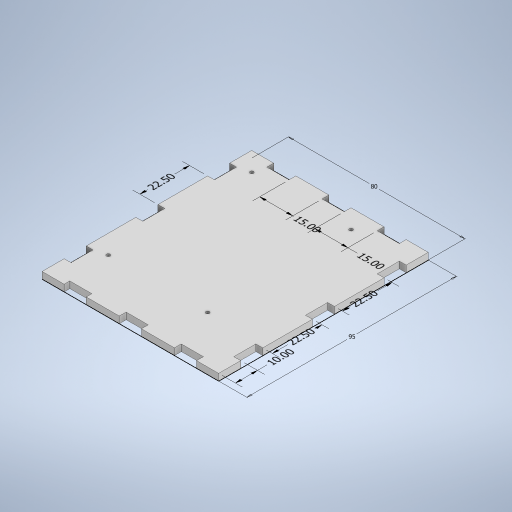
# Autodesk Inventor part: Fundo
Saved by Autodesk Inventor 2024 (Build 280153000, 153)
## iProperties
Created: 2023-11-29
Part Number: Fundo
Material: Genérico
Document SubType Name: Modeling
Designer: caiot
Density: 1 g/cm^3
Appearance: Padrão
Author: caiot
Autodesk Inventor part; units mm, degrees
ref_plane "YZ Plane" through (0, 0, 0) normal (1, 0, 0) x (0, 1, 0)
ref_plane "XZ Plane" through (0, 0, 0) normal (0, 1, 0) x (-1, 0, 0)
ref_plane "XY Plane" through (0, 0, 0) normal (0, 0, 1) x (1, 0, 0)
sketch "Fundo" plane through (0, 0, 0) normal (0, 1, 0) x (-1, 0, 0)
  line L0 (0, 0) -> (-80, 0)
  line L1 (-80, 0) -> (-80, -95)
  line L2 (-80, -95) -> (0, -95)
  line L3 (0, -95) -> (0, 0)
  dimension "d0" = 80
  dimension "d1" = 95
  constraints: 8 end point, 2 parallel, 1 horizontal, 1 perpendicular
  measures "d0" distance of L2.end L1.end
  measures "d1" distance of L1.end L0.end
extrude "Extrusão1" add sketch "Fundo" along normal blind 3
sketch "Esboço3" plane through (0, 3, 0) normal (0, 1, 0) x (1, 0, 0)
  line L0 (10, -0.55) -> (20, -0.55)
  line L1 (20, -0.55) -> (20, 2.55)
  line L2 (20, 2.55) -> (10, 2.55)
  line L3 (10, 2.55) -> (10, -0.55)
  line L4 (0, 0) -> (80, 0) projected
  line L5 (70, 0) -> (60, 0)
  line L6 (60, 0) -> (60, 3.1)
  line L7 (60, 3.1) -> (70, 3.1)
  line L8 (70, 3.1) -> (70, 0)
  line L9 (35, 0) -> (45, 0)
  line L10 (45, 0) -> (45, 3.1)
  line L11 (45, 3.1) -> (35, 3.1)
  line L12 (35, 3.1) -> (35, 0)
  line L13 (80, 95) -> (0, 95) projected
  line L14 (10, 95) -> (20, 95)
  line L15 (20, 95) -> (20, 91.9)
  line L16 (20, 91.9) -> (10, 91.9)
  line L17 (10, 91.9) -> (10, 95)
  line L18 (35, 95) -> (45, 95)
  line L19 (45, 95) -> (45, 91.9)
  line L20 (45, 91.9) -> (35, 91.9)
  line L21 (35, 91.9) -> (35, 95)
  line L22 (60, 95) -> (70, 95)
  line L23 (70, 95) -> (70, 91.9)
  line L24 (70, 91.9) -> (60, 91.9)
  line L25 (60, 91.9) -> (60, 95)
  line L26 (80, 0) -> (80, 95) projected
  line L27 (0, 95) -> (0, 0) projected
  point P0 (10, 1)
  point P1 (60, 1.55)
  point P2 (20, 1)
  point P3 (35, 1.55)
  point P4 (10, 93.45)
  point P5 (70, 93.45)
  point P6 (60, 93.45)
  point P7 (45, 93.45)
  point P8 (45, 1.55)
  point P9 (35, 93.45)
  point P10 (20, 93.45)
  point P11 (20, 95)
  point P12 (45, 0)
  point P13 (60, 0)
  point P14 (70, 1.55)
  dimension "d4" = 10
  dimension "d5" = 3.1
  dimension "d7" = 10
  dimension "d8" = 3.1
  dimension "d10" = 10
  dimension "d11" = 3.1
  dimension "d18" = 10
  dimension "d19" = 3.1
  dimension "d20" = 10
  dimension "d21" = 3.1
  dimension "d22" = 10
  dimension "d23" = 3.1
  dimension "d30" = 10
  dimension "d113" = 10
  dimension "d114" = 10
  dimension "d115" = 15
  dimension "d116" = 15
  dimension "d117" = 40
  dimension "d118" = 15
  dimension "d119" = 15
  dimension "d120" = 10
  constraints: 48 end point, 12 midpoint, 12 parallel, 6 horizontal, 6 perpendicular, 3 point on line, 3 other
  measures "d4" distance of L2.end L1.end
  measures "d5" distance of L1.end L0.end
  measures "d7" distance of L6.end L7.end
  measures "d8" distance of L5.end L6.end
  measures "d10" distance of L11.end L10.end
  measures "d11" distance of L10.end L9.end
  measures "d18" distance of L15.end L16.end
  measures "d19" distance of L14.end L15.end
  measures "d20" distance of L19.end L20.end
  measures "d21" distance of L18.end L19.end
  measures "d22" distance of L23.end L24.end
  measures "d23" distance of L22.end L23.end
  measures "d30" horizontal distance of L13.end point (10, 93.45)
  measures "d113" distance from line of L26 point (70, 1.55)
  measures "d114" distance from line of L27 point (10, 1)
  measures "d115" horizontal distance of point (35, 1.55) point (20, 1)
  measures "d116" distance of point (60, 1.55) point (45, 1.55)
  measures "d117" horizontal distance of point (20, 1) L6.end
  measures "d118" distance of point (35, 93.45) point (20, 93.45)
  measures "d119" distance of point (60, 93.45) point (45, 93.45)
  measures "d120" distance from line of L26 point (70, 93.45)
extrude "Extrusão2" cut sketch "Esboço3" against normal blind 10 contours L3 L4 L1 L0 | L3 L2 L1 L4 | L12 L11 L10 L4 | L13 L15 L16 L17 | L6 L7 L8 L4 | L13 L19 L20 L21 | L13 L23 L24 L25
sketch "Esboço4" plane through (0, 3, 0) normal (0, 1, 0) x (1, 0, 0)
  line L0 (0, 95) -> (0, 0) projected
  line L1 (0, 10) -> (3.1, 10)
  line L2 (3.1, 10) -> (3.1, 20)
  line L3 (3.1, 20) -> (0, 20)
  line L4 (0, 20) -> (0, 10)
  line L5 (0, 85) -> (3.1, 85)
  line L6 (3.1, 85) -> (3.1, 75)
  line L7 (3.1, 75) -> (0, 75)
  line L8 (0, 75) -> (0, 85)
  line L9 (0, 42.5) -> (3.1, 42.5)
  line L10 (3.1, 42.5) -> (3.1, 52.5)
  line L11 (3.1, 52.5) -> (0, 52.5)
  line L12 (0, 52.5) -> (0, 42.5)
  line L13 (10, 95) -> (0, 95) projected
  line L14 (80, 0) -> (80, 95) projected
  line L15 (80, 10) -> (76.9, 10)
  line L16 (76.9, 10) -> (76.9, 20)
  line L17 (76.9, 20) -> (80, 20)
  line L18 (80, 20) -> (80, 10)
  line L19 (80, 42.5) -> (76.9, 42.5)
  line L20 (76.9, 42.5) -> (76.9, 52.5)
  line L21 (76.9, 52.5) -> (80, 52.5)
  line L22 (80, 52.5) -> (80, 42.5)
  line L23 (80, 75) -> (76.9, 75)
  line L24 (76.9, 75) -> (76.9, 85)
  line L25 (76.9, 85) -> (80, 85)
  line L26 (80, 85) -> (80, 75)
  line L27 (70, 0) -> (80, 0) projected
  line L28 (80, 95) -> (70, 95) projected
  point P0 (1.55, 10)
  point P1 (1.55, 85)
  point P2 (1.55, 75)
  point P3 (1.55, 52.5)
  point P4 (1.55, 20)
  point P5 (78.45, 10)
  point P6 (78.45, 85)
  point P7 (78.45, 52.5)
  point P8 (78.45, 75)
  point P9 (80, 85)
  point P10 (0, 75)
  point P11 (0, 52.5)
  point P12 (0, 20)
  point P13 (78.45, 42.5)
  point P14 (78.45, 20)
  dimension "d44" = 3.1
  dimension "d45" = 10
  dimension "d46" = 10
  dimension "d47" = 3.1
  dimension "d48" = 10
  dimension "d49" = 10
  dimension "d50" = 10
  dimension "d51" = 22.5
  dimension "d53" = 3.1
  dimension "d54" = 10
  dimension "d55" = 3.1
  dimension "d56" = 10
  dimension "d57" = 3.1
  dimension "d58" = 10
  dimension "d59" = 10
  dimension "d60" = 10
  dimension "d61" = 22.5
  dimension "d64" = 22.5
  dimension "d130" = 55
  constraints: 48 end point, 12 parallel, 11 midpoint, 7 point on line, 6 horizontal, 6 perpendicular
  measures "d44" distance of L3.end L2.end
  measures "d45" distance of L2.end L1.end
  measures "d46" distance of L5.end L6.end
  measures "d47" distance of L11.end L10.end
  measures "d48" distance of L10.end L9.end
  measures "d49" vertical distance of L0.end point (1.55, 10)
  measures "d50" distance from line of L13 point (1.55, 85)
  measures "d51" distance of point (1.55, 75) point (1.55, 52.5)
  measures "d53" distance of L16.end L17.end
  measures "d54" distance of L15.end L16.end
  measures "d55" distance of L20.end L21.end
  measures "d56" distance of L19.end L20.end
  measures "d57" distance of L24.end L25.end
  measures "d58" distance of L23.end L24.end
  measures "d59" distance from line of L27 point (78.45, 10)
  measures "d60" distance from line of point (78.45, 85) L28
  measures "d61" distance of point (78.45, 52.5) point (78.45, 75)
  measures "d64" distance of point (78.45, 42.5) point (78.45, 20)
  measures "d130" distance of point (78.45, 20) point (78.45, 75)
extrude "Extrusão3" cut sketch "Esboço4" against normal blind 10
sketch "Esboço6" plane through (0, 3, 0) normal (0, 1, 0) x (1, 0, 0)
  line L0 (8.6, 86.4) -> (53.6, 86.4)
  line L1 (53.6, 86.4) -> (53.6, 21.4)
  line L2 (53.6, 21.4) -> (8.6, 21.4)
  line L3 (8.6, 21.4) -> (8.6, 86.4)
  line L4 (3.1, 85) -> (3.1, 75) projected
  line L5 (20, 91.9) -> (10, 91.9) projected
  circle A0 centre (53.6, 86.4) radius 0.8
  circle A1 centre (53.6, 21.4) radius 0.8
  circle A2 centre (8.6, 21.4) radius 0.8
  circle A3 centre (8.6, 86.4) radius 0.8
  point P0 (0, 0)
  point P1 (3.1, 80)
  point P2 (15, 91.9)
  dimension "d134" = 65
  dimension "d135" = 45
  dimension "d136" = 5.5
  dimension "d137" = 5.5
  dimension "d138" = 1.6
  dimension "d139" = 1.6
  dimension "d140" = 1.6
  dimension "d141" = 1.6
  constraints: 8 end point, 4 centre point, 4 coincident, 2 midpoint, 2 parallel, 1 horizontal, 1 perpendicular
  measures "d134" distance of L0.end L1.end
  measures "d135" distance between parallel lines of L3 L1
  measures "d136" distance from line of point (3.1, 80) L3
  measures "d137" distance from line of point (15, 91.9) L0
  measures "d138" diameter of A0
  measures "d139" diameter of A1
  measures "d140" diameter of A2
  measures "d141" diameter of A3
extrude "Extrusão4" cut sketch "Esboço6" against normal blind 10 contours L3 A3 L0 | L0 A3 L3 | A0 L1 L0 | L0 L1 A0 | A2 L2 L3 | L3 L2 A2 | A1 L2 L1 | L1 L2 A1
